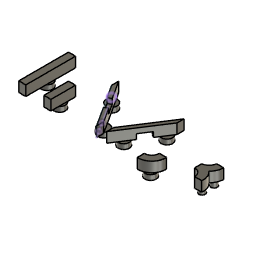
Segments v5 (Autodesk Fusion 360 design; units mm, degrees)
Autodesk Fusion 360 part; units mm, degrees
sketch "Skizze1" plane through (0, 0, 0) normal (0, 0, 1) x (1, 0, 0)
  line L0 (0, 0) -> (2.8, 0)
  line L1 (2.8, 0) -> (2.8, 19.8)
  line L2 (2.8, 19.8) -> (0, 19.8)
  line L3 (0, 19.8) -> (0, 0)
  line L4 (10, 0) -> (12.8, 0)
  line L5 (12.8, 0) -> (12.8, 9.8)
  line L6 (12.8, 9.8) -> (10, 9.8)
  line L7 (10, 9.8) -> (10, 0)
  circle A0 centre (11.4, 4.9) radius 2.25
  circle A1 centre (1.4, 9.9) radius 2.25
  line L8 (1.4, 19.8) -> (1.4, 9.9)
  line L9 (20, 19.8) -> (20, 17)
  line L10 (31, 0) -> (31, 2.8)
  line L11 (31, 2.8) -> (20, 19.8)
  line L12 (20, 17) -> (31, 0)
  line L13 (35, 0) -> (35, 2.8)
  line L14 (35, 2.8) -> (46, 19.8)
  line L15 (46, 19.8) -> (46, 17)
  line L16 (46, 17) -> (35, 0)
  line L17 (50, 0) -> (50, -2.8)
  line L18 (53, 2.999) -> (55.8, 2.999)
  arc A2 (50, 0) -> (53, 2.999) centre (50.0962, 2.9038) ccw
  arc A3 (50, -2.8) -> (55.8, 2.999) centre (50.3035, 2.6965) ccw
  line L19 (50, 0) -> (50, -0.5)
  line L20 (50, -0.5) -> (53, -0.5)
  circle A4 centre (53, -0.5) radius 2.25
  line L21 (46, 17) -> (46, 15)
  line L22 (46, 15) -> (44, 15)
  circle A5 centre (44, 15) radius 2.25
  line L23 (20, 17) -> (20, 15)
  line L24 (65, 5) -> (65, 7.8)
  line L25 (65, 7.8) -> (65, 10.8)
  line L26 (65, 10.8) -> (68, 10.8)
  line L27 (68, 10.8) -> (70.8, 10.8)
  arc A6 (65, 7.8) -> (68, 10.8) centre (64.5, 11.3) ccw
  arc A7 (65, 5) -> (70.8, 10.8) centre (64.8369, 10.9631) ccw
  line L28 (65, 5) -> (65, 2)
  line L29 (65, 2) -> (68, 2)
  line L30 (68, 2) -> (70.8, 2)
  arc A8 (68, 2) -> (65, 5) centre (65.0799, 2.0799) ccw
  arc A9 (70.8, 2) -> (65, 7.8) centre (65.725, 2.725) ccw
  line L31 (68, 10.8) -> (69, 10.8)
  line L32 (69, 10.8) -> (69, 8.8)
  circle A10 centre (69, 8.8) radius 1.25
  line L33 (69.0147, 2) -> (69.0147, 4)
  circle A11 centre (69.0147, 4) radius 1.25
  line L34 (65, 7.8) -> (65, 6.3)
  line L35 (65, 6.3) -> (66.5, 6.3)
  circle A12 centre (66.5, 6.3) radius 1.25
  line L36 (46, 17) -> (41.4704, 9.9997)
  line L37 (41.4704, 9.9997) -> (40.1933, 10.826)
  line L38 (41.4704, 9.9997) -> (40.4996, 8.4994)
  line L39 (40.4996, 8.4994) -> (39.2225, 9.3257)
  line L40 (20, 17) -> (24.5296, 9.9997)
  line L41 (20, 19.8) -> (25.4999, 11.3002)
  line L42 (25.4999, 11.3002) -> (24.5296, 9.9997)
  line L43 (25.4999, 11.3002) -> (26.4707, 9.7999)
  line L44 (24.5296, 9.9997) -> (25.5004, 8.4994)
  line L45 (25.5004, 8.4994) -> (26.4707, 9.7999)
  line L46 (31, 2.8) -> (31, 4.8)
  line L47 (31, 4.8) -> (29, 4.8)
  circle A13 centre (22, 15) radius 2.25
  line L48 (22, 15) -> (20, 15)
  circle A14 centre (29, 4.8) radius 2.25
  line L49 (35, 2.8) -> (35, 4.8)
  line L50 (35, 4.8) -> (37, 4.8)
  circle A15 centre (37, 4.8) radius 2.25
  dimension "d1" = 2.8
  dimension "d2" = 19.8
  dimension "d3" = 2.8
  dimension "d4" = 9.8
  dimension "d5" = 4.5
  dimension "d6" = 4.5
  dimension "d9" = 2.8
  dimension "d10" = 2.8
  dimension "d11" = 9.9
  dimension "d14" = 2.8
  dimension "d15" = 0.5
  dimension "d16" = 3
  dimension "d17" = 4.5
  dimension "d18" = 2.8
  dimension "d19" = 2
  dimension "d20" = 4.5
  dimension "d22" = 2.8
  dimension "d23" = 3
  dimension "d24" = 3
  dimension "d25" = 2.8
  dimension "d26" = 3
  dimension "d27" = 3
  dimension "d28" = 2.8
  dimension "d29" = 1
  dimension "d30" = 2
  dimension "d31" = 2.5
  dimension "d32" = 2
  dimension "d33" = 2.5
  dimension "d34" = 1.5
  dimension "d35" = 1.5
  dimension "d36" = 2.5
  dimension "d41" = 8.338
  dimension "d42" = 1.787
  dimension "d47" = 8.338
  dimension "d48" = 10.124
  dimension "d49" = 1.787
  dimension "d50" = 1.787
  dimension "d56" = 2
  dimension "d57" = 2
  dimension "d58" = 4.5
  dimension "d59" = 4.5
  dimension "d60" = 2
  dimension "d61" = 2
  dimension "d62" = 4.5
  constraint horizontal L0
  constraint vertical L1
  constraint horizontal L2
  constraint vertical L3
  constraint coincident L0.start L3.end
  constraint horizontal L4
  constraint vertical L5
  constraint horizontal L6
  constraint vertical L7
  constraint midpoint L2 L8.start
  constraint perpendicular L0 L8
  constraint coincident A1.centre L8.end
  constraint vertical L9
  constraint vertical L13
  constraint parallel L13 L15
  constraint parallel L14 L16
  constraint coincident L17 L19.end
  constraint horizontal L20
  constraint coincident L20.end A4.centre
  constraint parallel L15 L21
  constraint perpendicular L21 L22
  constraint coincident L22.end A5.centre
  constraint parallel L9 L23
  constraint vertical L24
  constraint parallel L24 L25
  constraint perpendicular L25 L26
  constraint perpendicular L25 L27
  constraint parallel L24 L28
  constraint perpendicular L28 L29
  constraint perpendicular L28 L30
  constraint tangent A7 A8
  constraint tangent A6 A9
  constraint parallel L27 L31
  constraint perpendicular L31 L32
  constraint coincident L32.end A10.centre
  constraint coincident L30 L33.start
  constraint perpendicular L30 L33
  constraint coincident L33.end A11.centre
  constraint coincident L24 L34.end
  constraint perpendicular L34 L35
  constraint coincident L35.end A12.centre
  constraint coincident L16 L36.end
  constraint coincident L14 L37.end
  constraint perpendicular L14 L37
  constraint coincident L16 L38.end
  constraint coincident L14 L39.end
  constraint perpendicular L14 L39
  constraint coincident L12 L40.end
  constraint coincident L11 L41.end
  constraint coincident L11 L43.end
  constraint coincident L12 L44.end
  constraint parallel L10 L46
  constraint perpendicular L46 L47
  constraint coincident A13.centre L48.start
  constraint perpendicular L23 L48
  constraint coincident L47.end A14.centre
  constraint parallel L13 L49
  constraint perpendicular L49 L50
  constraint coincident L50.end A15.centre
  measures "d1" distance of L0.start L0.end
  measures "d2" distance of L0.start L2.end
  measures "d3" distance of L4.start L4.end
  measures "d4" distance of L4.start L6.end
  measures "d5" diameter of A0
  measures "d6" diameter of A1
  measures "d9" distance of L10.start L10.end
  measures "d10" distance of L13.start L13.end
  measures "d11" distance of L8.start A1.centre
  measures "d14" distance of L18.start L18.end
  measures "d15" distance of L17.start L19.end
  measures "d16" distance of L19.end L20.end
  measures "d17" diameter of A4
  measures "d18" distance of L17.start L17.end
  measures "d19" distance of L21.end L22.end
  measures "d20" diameter of A5
  measures "d22" distance of L24.start L24.end
  measures "d23" distance of L24.end L25.end
  measures "d24" distance of L25.end L26.end
  measures "d25" distance of L26.end L27.end
  measures "d26" distance of L24.start L28.end
  measures "d27" distance of L28.end L29.end
  measures "d28" distance of L29.end L30.end
  measures "d29" distance of L26.end L31.end
  measures "d30" distance of L31.end L32.end
  measures "d31" diameter of A10
  measures "d32" distance of L33.start L33.end
  measures "d33" diameter of A11
  measures "d34" distance of L24.end L34.end
  measures "d35" distance of L34.end L35.end
  measures "d36" diameter of A12
  measures "d41" distance of L15.end L36.end
  measures "d42" distance of L36.end L38.end
  measures "d47" distance of L9.end L40.end
  measures "d48" distance of L9.start L41.end
  measures "d49" distance of L41.end L43.end
  measures "d50" distance of L40.end L44.end
  measures "d56" distance of L10.end L46.end
  measures "d57" distance of L46.end L47.end
  measures "d58" diameter of A13
  measures "d59" diameter of A14
  measures "d60" distance of L13.end L49.end
  measures "d61" distance of L49.end L50.end
  measures "d62" diameter of A15
extrude "Extrusion1" add sketch "Skizze1" along normal blind 4 contours L0 L1 L3 A1 | L1 L3 A1 | L2 L3 A1 L8 | L1 L2 A1 L8 | L4 L5 L7 A0 | L5 L7 A0 | L5 L6 L7 A0 | L9 L11 L12 L40 L41 A13 | L11 L12 L40 L41 A13 | L11 L12 L40 L41 L42 A13 | L11 L12 L42 L43 L44 L45 | L11 L12 L45 A14 | L11 L12 A14 | L10 L11 L12 A14 | L13 L14 L16 A15 | L14 L16 A15 | L14 L16 L39 A15 | L14 L16 L37 L38 L39 | L14 L16 A5 L36 L37 | L14 L16 A5 L36 | L14 L15 L16 A5 L36 | L17 A2 L19 L20 A4 | L17 A3 L20 A4 | A2 A3 A4 | L18 A2 A3 A4 | L24 A7 L35 A12 | A7 L30 A8 A9 A12 | L24 A7 A9 L34 L35 A12 | A7 A12 | A7 A12 | L27 A6 A7 A9 L31 | A10 | A11 makes body 1 at (38.6667, 8.4667, 2.6667) makes body 2 at (0, 13.2, 1.3333) makes body 3 at (53.8157, -1.5424, 2.6667) makes body 4 at (27.3333, 8.4667, 1.3333) makes body 5 at (10, 6.5333, 1.3333) makes body 6 at (67.0718, 6.5047, 0)
extrude "Extrusion2" add sketch "Skizze1" against normal blind 2 contours L3 A1 | L1 L3 A1 | L1 A1 | L7 A0 | L5 L7 A0 | L5 A0 | L11 L41 A13 | L11 L12 L40 L41 A13 | L12 L23 L40 A13 L48 | L12 L23 L40 A13 L48 | L11 L46 L47 A14 | L11 L12 A14 | L12 A14 | L11 L46 L47 A14 | L14 L16 A15 | L16 A15 | L14 L49 L50 A15 | L14 L49 L50 A15 | L14 L16 A5 L36 | L16 L21 L22 A5 L36 | L14 A5 | L16 L21 L22 A5 L36 | A2 A4 | A2 A3 A4 | A3 A4 | A7 A12 | A7 A12 | A10 | A11 bodies 6 3 1 4 5 2
sketch "Skizze2" plane through (21.8512, 14.139, 0) normal (-0.83957, -0.543251, 0) x (0.543251, -0.83957, 0)
  line L0 (-3.4077, 0) -> (-2.8126, 0)
  line L1 (-2.8126, 0) -> (1.5285, 0)
  line L2 (16.8408, 0) -> (16.8408, 4)
  line L3 (16.8408, 4) -> (-3.4077, 4)
  line L4 (-3.4077, 4) -> (-3.4077, 0)
  line L5 (1.5285, 0) -> (9.6749, 0)
  line L6 (9.6749, 0) -> (13.7739, 0)
  line L7 (13.7739, 0) -> (16.8408, 0)
sketch "Skizze3" plane through (24.6707, -15.9634, 0) normal (0.83957, -0.543251, 0) x (0.543251, 0.83957, 0)
  line L0 (38.6672, 0) -> (39.2623, 0)
  line L1 (39.2623, 0) -> (39.2623, 4)
  line L2 (39.2623, 4) -> (19.0138, 4)
  line L3 (19.0138, 4) -> (19.0138, 0)
  line L4 (26.1797, 0) -> (34.3261, 0)
  line L5 (22.0807, 0) -> (26.1797, 0)
  line L6 (32.5, 0) -> (27.6, 0)
  line L7 (27.6, 0) -> (27.6, 2)
  line L8 (27.6, 2) -> (32.5, 2)
  line L9 (32.5, 2) -> (32.5, 0)
  line L10 (19.0138, 0) -> (22.0807, 0)
  line L11 (34.3261, 0) -> (38.6672, 0)
  dimension "d43" = 4.9
  dimension "d44" = 2
  constraint horizontal L6
  constraint vertical L7
  constraint horizontal L8
  constraint vertical L9
  constraint coincident L4 L6.start
  measures "d43" distance of L6.start L6.end
  measures "d44" distance of L6.start L8.end
extrude "Extrusion3" cut sketch "Skizze3" against normal blind 1.6 contours L4 L6 L7 L8 L9 bodies 1
sketch "Skizze4" plane through (23.1283, 14.9654, 0) normal (0.83957, 0.543251, 0) x (-0.543251, 0.83957, 0)
  line L0 (-14.49, 0) -> (-13.8949, 0)
  line L1 (5.7585, 0) -> (5.7585, 4)
  line L2 (5.7585, 4) -> (-14.49, 4)
  line L3 (-14.49, 4) -> (-14.49, 0)
  line L4 (-4.36, 0) -> (-4.36, 2)
  line L5 (-4.36, 2) -> (-6.15, 2)
  line L6 (-6.15, 0) -> (-6.15, 2)
  line L7 (-4.36, 2) -> (-2.86, 2)
  line L8 (-2.86, 2) -> (-2.86, 4)
  line L9 (-2.86, 4) -> (-4.36, 4)
  line L10 (-4.36, 4) -> (-4.36, 2)
  line L11 (-4.36, 2) -> (-6.15, 2)
  line L12 (-6.15, 2) -> (-6.15, 4)
  line L13 (-6.15, 4) -> (-4.36, 4)
  line L14 (-4.36, 4) -> (-4.36, 2)
  line L15 (-6.15, 2) -> (-7.65, 2)
  line L16 (-7.65, 2) -> (-7.65, 4)
  line L17 (-7.65, 4) -> (-6.15, 4)
  line L18 (-6.15, 4) -> (-6.15, 2)
  line L19 (-13.8949, 0) -> (-9.5538, 0)
  line L20 (-9.5538, 0) -> (-1.4075, 0)
  line L21 (-1.4075, 0) -> (2.6915, 0)
  line L22 (2.6915, 0) -> (5.7585, 0)
  dimension "d51" = 2
  dimension "d52" = 1.5
  dimension "d53" = 1.5
  constraint coincident L0 L4.start
  constraint perpendicular L2 L4
  constraint perpendicular L4 L5
  constraint coincident L0 L6.start
  constraint perpendicular L5 L6
  constraint horizontal L7
  constraint vertical L8
  constraint horizontal L9
  constraint vertical L10
  constraint coincident L2 L8.end
  constraint horizontal L11
  constraint vertical L12
  constraint horizontal L13
  constraint vertical L14
  constraint coincident L2 L12.end
  constraint horizontal L15
  constraint vertical L16
  constraint horizontal L17
  constraint vertical L18
  constraint coincident L2 L16.end
  measures "d51" distance of L4.start L4.end
  measures "d52" distance of L4.end L7.end
  measures "d53" distance of L5.end L15.end
extrude "Extrusion4" cut sketch "Skizze4" against normal blind 2.5 contours L2 L12 L15 L16 L17 L18 | L2 L5 L10 L11 L12 L13 L14 L18 | L2 L7 L8 L9 L10 L14 bodies 4
copy_body "Körper->Berechn1" bodies 2 removing the originals makes body 7 in component "Segment lang"
copy_body "Körper->Berechn2" bodies 5 removing the originals makes body 8 in component "Segment Kurz"
copy_body "Körper->Berechn3" bodies 4 removing the originals makes body 9 in component "Schraeges Segment 1"
copy_body "Körper->Berechn4" bodies 1 removing the originals makes body 10 in component "Schraeges Segment2"
copy_body "Körper->Berechn5" bodies 3 removing the originals makes body 11 in component "Rundes Segment"
copy_body "Körper->Berechn6" bodies 6 removing the originals makes body 12 in component "Rundes Segment doppelt"
component "Segment lang" placed x (1, 0, 0) y (0, 1, 0) z (0, 0, 1) at (0, 0, 0)
component "Segment Kurz" placed x (1, 0, 0) y (0, 1, 0) z (0, 0, 1) at (0, 0, 0)
component "Schraeges Segment 1" placed x (1, 0, 0) y (0, 1, 0) z (0, 0, 1) at (0, 0, 0)
component "Schraeges Segment2" placed x (1, 0, 0) y (0, 1, 0) z (0, 0, 1) at (0, 0, 0)
component "Rundes Segment" placed x (1, 0, 0) y (0, 1, 0) z (0, 0, 1) at (0, 0, 0)
component "Rundes Segment doppelt" placed x (1, 0, 0) y (0, 1, 0) z (0, 0, 1) at (0, 0, 0)
